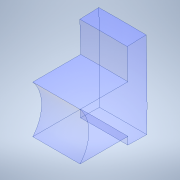
# Autodesk Inventor part: shank_2
Saved by Autodesk Inventor 2020.2 (Build 242310000, 310)
## iProperties
Created: 2021-01-30
Part Number: shank_2
Material: Generic
Document SubType Name: Modeling
Designer: DELL
Density: 1 g/cm^3
Appearance: Clear - Blue
Author: DELL
Autodesk Inventor part; units mm, degrees
ref_plane "XZ Plane" through (0, 0, 0) normal (0, 1, 0) x (-1, 0, 0)
ref_plane "XY Plane" through (0, 0, 0) normal (0, 0, 1) x (1, 0, 0)
ref_plane "UCS1: YZ Plane" through (0, 0, 0) normal (1, 0, 0) x (0, 1, 0)
sketch "Sketch17" plane through (0, 0, 0) normal (1, 0, 0) x (0, 1, 0)
  line L0 (-76.0002, 0) -> (106.0011, 0) construction
  line L1 (0, -525.3205) -> (0, 2308.9037) projected
  circle A0 centre (0, 0) radius 40
  circle A1 centre (0, 0) radius 46
  arc A2 (-49.3998, -95.3753) -> (79.0446, -94.4228) centre (0, 1904.0145) ccw
  arc A3 (-50, -119.3749) -> (79.993, -118.3996) centre (0, 1880) ccw
  line L2 (79.0446, -94.4228) -> (79.993, -118.3996)
  line L3 (-50, -119.3749) -> (-49.3998, -95.3753)
  line L4 (-30, -34.8712) -> (-30, -95.9855)
  line L5 (-30, -95.9855) -> (30, -95.9855)
  line L6 (30, -95.9855) -> (30, -34.8712)
  line L7 (-39.5198, -95.595) -> (-40, -119.6)
  line L8 (69.16, -94.7893) -> (70, -118.7746)
  line L9 (36.9845, -80.3466) -> (53.2471, -80.3466) construction
  line L10 (53.2471, -80.3466) -> (53.2471, -83.7318) construction
  line L11 (53.2471, -83.7318) -> (36.9845, -83.7318) construction
  line L12 (36.9845, -83.7318) -> (36.9845, -80.3466) construction
  point P0 (0, -120.0626)
  point P1 (0, -95.9855)
  point P2 (0, -46)
  point P3 (0, -95.9855)
  point P4 (30, -95.7605)
  point P5 (0, -95.9855)
  point P6 (-30, -95.7605)
  point P7 (0, -120)
  dimension "d173" = 92
  dimension "d174" = 80
  dimension "d224" = 60
  dimension "d230" = 2000
  dimension "d231" = 23.9956
  dimension "d233" = 10
  dimension "d235" = 2000
  dimension "d241" = 24
  dimension "d246" = 40
  dimension "d247" = 70
  dimension "d248" = 10
  dimension "d249" = 120
  constraints: 14 end point, 12 point on circle, 4 centre point, 4 line through centre, 3 point on line, 2 coincident, 2 perpendicular, 1 tangent, 1 vertical, 3 other
  measures "d173" diameter of A1
  measures "d174" diameter of A0
  measures "d224" distance of L4.end L5.end
  measures "d230" radius of A3
  measures "d231" distance of L2.start L2.end
  measures "d233" horizontal distance of L3.start L7.end
  measures "d235" radius of A2
  measures "d241" distance of L8.start L8.end
  measures "d246" distance from line of L7.end L1
  measures "d247" distance from line of L8.end L1
  measures "d248" distance of L2.end L8.end
  measures "d249" distance from line of point (0, -120) L0
revolve "Revolution2" add sketch "Sketch17" angle 360 about axis through (0, 0, -10) along (0, 0, 1) contours L1 L5 L6 A2 L8 A3 | A2 L6 L5 | L8 A2 L2 A3
ref_plane "Work Plane7" through (0, -39.5198, -95.595) normal (0, -0.9998, 0.02) x (0, -0.02, -0.9998)
split "Split2" plane through (0, -39.5198, -95.595) removes the side toward (0, -0.9998, 0.02)
ref_plane "Work Plane8" through (0, 69.16, -94.7893) normal (0, -0.9993873, -0.035) x (0, 0.035, -0.9993873)
split "Split3" plane through (0, 69.16, -94.7893) removes the side toward (0, 0.9993873, 0.035)
ref_plane "Work Plane9" through (-30, 0, 0) normal (1, 0, 0) x (0, 1, 0)
split "Split4" plane through (-30, 0, 0) removes the side toward (-1, 0, 0)
ref_plane "Work Plane10" through (30, 0, 0) normal (1, 0, 0) x (0, 1, 0)
split "Split5" plane through (30, 0, 0) removes the side toward (1, 0, 0)
extrude "Extrusion17" add sketch "Sketch17" along normal mid plane 60 contours L1 A1 L6 A2 | A2 L6 L5
fillet "Fillet16" [suppressed]
mirror "Mirror4" about plane through (0, 0, 0) normal (0, 1, 0) of "Extrusion17"
body "Solid1"
body "Solid8"
